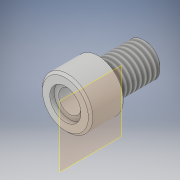
# Autodesk Inventor part: shaftSealBulkhead
Saved by Autodesk Inventor 2018 (Build 220112000, 112)
## iProperties
Created: 2020-02-25
Part Number: shaftSealBulkhead
Material: Generic
Document SubType Name: Modeling
Designer: anirudh
Density: 1 g/cm^3
Appearance: Default
Author: anirudh
Autodesk Inventor part; units mm, degrees
ref_plane "YZ Plane" through (0, 0, 0) normal (1, 0, 0) x (0, 1, 0)
ref_plane "XZ Plane" through (0, 0, 0) normal (0, 1, 0) x (-1, 0, 0)
ref_plane "XY Plane" through (0, 0, 0) normal (0, 0, 1) x (1, 0, 0)
sketch "Sketch1" plane through (0, 0, 0) normal (0, 0, 1) x (1, 0, 0)
  circle A0 centre (0, 0) radius 9
  dimension "d0" = 18
  constraints: 1 centre point, 1 coincident
  measures "d0" diameter of A0
extrude "Extrusion1" add sketch "Sketch1" against normal blind 12
sketch "Sketch2" plane through (0, 0, -12) normal (0, 0, -1) x (-1, 0, 0)
  circle A0 centre (0, 0) radius 5.9688
  constraints: 1 centre point, 1 coincident
extrude "Extrusion2" add sketch "Sketch2" along normal blind 16.5862
sketch "Sketch3" plane through (0, 0, -12) normal (0, 0, -1) x (-1, 0, 0)
  circle A0 centre (0, 0) radius 5.41
  circle A1 centre (0, 0) radius 6.41
  circle A2 centre (0, 0) radius 8
  dimension "d7" = 10.82
  dimension "d29" = 12.82
  dimension "d30" = 16
  constraints: 3 centre point, 2 coincident
  measures "d7" diameter of A0
  measures "d29" diameter of A1
  measures "d30" diameter of A2
sketch "Sketch4" plane through (0, 0, -28.5862) normal (0, 0, -1) x (-1, 0, 0)
  circle A0 centre (0, 0) radius 3.9688
  dimension "d13" = 7.9375
  constraints: 1 centre point, 1 coincident
  measures "d13" diameter of A0
extrude "Extrusion4" cut sketch "Sketch4" against normal blind 36.5125
sketch "Sketch5" plane through (0, 0, 0) normal (0, 0, 1) x (1, 0, 0)
  circle A0 centre (0, 0) radius 5.5563
  dimension "d16" = 11.1125
  constraints: 1 centre point, 1 coincident
  measures "d16" diameter of A0
extrude "Extrusion5" cut sketch "Sketch5" against normal blind 1.5875
sketch "Sketch6" plane through (0, 0, -28.5862) normal (0, 0, -1) x (-1, 0, 0)
  circle A0 centre (0, 0) radius 6
  circle A1 centre (0, 0) radius 5.9687
  dimension "d19" = 12
  constraints: 2 centre point, 2 coincident
  measures "d19" diameter of A0
extrude "Extrusion6" add sketch "Sketch6" against normal blind 16.5862
chamfer "Chamfer1" distance 0.7937 angle 45 1 edges at (-9, 0, 0)
chamfer "Chamfer2" distance 0.7937 angle 45 1 edges at (6, 0, -28.5862)
sketch "Sketch7" plane through (0, 0, -12) normal (0, 0, -1) x (-1, 0, 0)
  arc A0 (0, -9) -> (0, 9) centre (0, 0) ccw
  line L0 (9, 0) -> (9, 13.6838)
  arc A1 (0, 9.6783) -> (0, -9.6783) centre (0, 0) ccw
  line L1 (0, -9.6783) -> (0, -9)
  line L2 (0, 9) -> (0, 9.6783)
  constraints: 6 end point, 4 point on circle, 3 vertical, 2 centre point, 2 coincident
revolve "Revolution1" cut sketch "Sketch7" angle 1 about axis through (-9, 0, -12) along (0, -1, 0)
sketch "Sketch8" plane through (0, 0, -12) normal (0, 0, 1) x (1, 0, 0)
  circle A0 centre (0, 0) radius 3.9687
  circle A1 centre (0, 0) radius 6
  constraints: 2 centre point, 2 coincident
extrude "Extrusion8" add sketch "Sketch8" along normal blind 1.25
sketch "Sketch9" plane through (0, 0, -11.8429) normal (0.0174524, 0, -0.9998477) x (-0.9998477, 0, -0.0174524)
  circle A0 centre (0, 0) radius 6.41
  circle A1 centre (0, 0) radius 8
  dimension "d40" = 12.82
  dimension "d41" = 16
  constraints: 2 centre point, 1 coincident
  measures "d40" diameter of A0
  measures "d41" diameter of A1
extrude "Extrusion9" cut sketch "Sketch9" against normal blind 1.25
thread "Thread2" size "M12x1.75" class "6g" standard "ANSI Metric M Profile" full length
sketch "Sketch11" plane through (0, 0, 0) normal (0, 0, 1) x (1, 0, 0)
  line L0 (0, 0) -> (9, 0)
  circle A0 centre (0, 0) radius 9 projected
  constraints: 2 end point, 1 horizontal, 1 horizontal alignment, 1 other
ref_plane "Work Plane2" through (9, 0, 0) normal (1, 0, 0) x (0, 1, 0)
body "Solid1"
